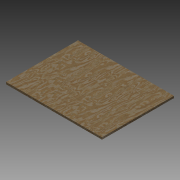
# Autodesk Inventor part: TopPlatform
Saved by Autodesk Inventor 2015 SP1 (Build 190203100, 203)
## iProperties
Created: 2016-02-22
Part Number: TopPlatform
Material: Generic
Document SubType Name: Modeling
Designer: Mac
Density: 1 g/cm^3
Appearance: Plywood - Weathered
Author: Mac
Autodesk Inventor part; units mm, degrees
ref_plane "YZ Plane" through (0, 0, 0) normal (1, 0, 0) x (0, 1, 0)
ref_plane "XZ Plane" through (0, 0, 0) normal (0, 1, 0) x (-1, 0, 0)
ref_plane "XY Plane" through (0, 0, 0) normal (0, 0, 1) x (1, 0, 0)
sketch "Sketch1" plane through (0, 0, 0) normal (0, 1, 0) x (-1, 0, 0)
  line L0 (609.6, 457.2) -> (-609.6, 457.2)
  line L1 (-609.6, 457.2) -> (-609.6, -457.2)
  line L2 (-609.6, -457.2) -> (609.6, -457.2)
  line L3 (609.6, -457.2) -> (609.6, 457.2)
  point P0 (0, 0)
  point P1 (609.6, 0)
  point P2 (0, -457.2)
  dimension "d0" = 914.4
  dimension "d1" = 1219.2
  constraints: 8 end point, 2 midpoint, 2 parallel, 1 horizontal, 1 horizontal alignment, 1 perpendicular, 1 vertical alignment
  measures "d0" distance of L2.end L0.start
  measures "d1" distance of L1.end L2.end
extrude "Extrusion1" add sketch "Sketch1" along normal blind 25.4
body "Solid1"
